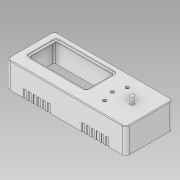
# Autodesk Inventor part: TAPA SUPEIOR
Saved by Autodesk Inventor 2019 (Build 230136000, 136)
## iProperties
Created: 2019-07-31
Part Number: TAPA SUPEIOR
Material: Plástico ABS
Document SubType Name: Modeling
Designer: Luis Pujol
Density: 1.06 g/cm^3
Appearance: Suave - Blanco
Author: Luis Pujol
Autodesk Inventor part; units mm, degrees
ref_plane "YZ Plane" through (0, 0, 0) normal (1, 0, 0) x (0, 1, 0)
ref_plane "XZ Plane" through (0, 0, 0) normal (0, 1, 0) x (-1, 0, 0)
ref_plane "XY Plane" through (0, 0, 0) normal (0, 0, 1) x (1, 0, 0)
sketch "Boceto1" plane through (0, 0, 0) normal (0, 1, 0) x (-1, 0, 0)
  line L0 (87.5, 35) -> (-87.5, 35)
  line L1 (-87.5, 35) -> (-87.5, -35)
  line L2 (-87.5, -35) -> (87.5, -35)
  line L3 (87.5, -35) -> (87.5, 35)
  line L4 (87.5, 35) -> (-87.5, -35) construction
  line L5 (-87.5, 35) -> (87.5, -35) construction
  point P0 (0, 0)
  dimension "d0" = 175
  dimension "d1" = 70
  constraints: 12 end point, 2 midpoint, 2 parallel, 1 horizontal, 1 perpendicular
  measures "d0" distance of L2.end L1.end
  measures "d1" distance of L1.end L0.end
extrude "Extrusión1" add sketch "Boceto1" along normal blind 2.8
fillet "Empalme1" radius 5 4 edges at (87.5, 1.4, 35) (87.5, 1.4, -35) (-87.5, 1.4, 35) (-87.5, 1.4, -35)
sketch "Boceto2" plane through (0, 0, 0) normal (0, -1, 0) x (1, 0, 0)
  arc A0 (-87.5, -30) -> (-82.5, -35) centre (-82.5, -30) ccw projected
  line L0 (82.5, -35) -> (-82.5, -35) projected
  arc A1 (82.5, -35) -> (87.5, -30) centre (82.5, -30) ccw projected
  line L1 (87.5, 30) -> (87.5, -30) projected
  arc A2 (87.5, 30) -> (82.5, 35) centre (82.5, 30) ccw projected
  line L2 (-82.5, 35) -> (82.5, 35) projected
  arc A3 (-82.5, 35) -> (-87.5, 30) centre (-82.5, 30) ccw projected
  line L3 (-87.5, -30) -> (-87.5, 30) projected
  arc A4 (84.7, 30) -> (82.5, 32.2) centre (82.5, 30) ccw
  line L4 (84.7, 30) -> (84.7, -30)
  arc A5 (82.5, -32.2) -> (84.7, -30) centre (82.5, -30) ccw
  line L5 (82.5, -32.2) -> (-82.5, -32.2)
  arc A6 (-84.7, -30) -> (-82.5, -32.2) centre (-82.5, -30) ccw
  line L6 (-84.7, -30) -> (-84.7, 30)
  arc A7 (-82.5, 32.2) -> (-84.7, 30) centre (-82.5, 30) ccw
  line L7 (-82.5, 32.2) -> (82.5, 32.2)
  point P0 (0, 0)
  dimension "d5" = 2.8
  constraints: 8 end point, 8 point on circle, 4 centre point, 7 other
  measures "d5" distance between parallel lines of L2 L7
extrude "Extrusión2" add sketch "Boceto2" along normal blind 35
sketch "Boceto8" plane through (0, 0, 0) normal (0, -1, 0) x (1, 0, 0)
  circle A0 centre (24.3039, 17.2337) radius 2.5
  point P0 (0, 0)
  dimension "d40" = 5
  constraints: 1 centre point
  measures "d40" diameter of A0
extrude "Extrusión8" add sketch "Boceto8" along normal blind 3.3
fillet "Empalme3" radius 0.5 2 edges at (21.8039, 0, 17.2337) (21.8039, -3.3, 17.2337)
sketch "Boceto11" plane through (24.3039, -3.3, 17.2337) normal (0, -1, 0) x (1, 0, 0)
  circle A0 centre (0, 0) radius 2 projected
  point P0 (-24.3039, -17.2337)
hole "Agujero2" at (24.3039, -3.3, 17.2337) direction (0, 1, 0) diameter 1.8 depth 5 tip angle 118 countersink diameter 2.5 countersink angle 90
fillet "Empalme4" radius 1 8 edges at (-86.0355, 2.8, 33.5355) (0, 2.8, 35) (86.0355, 2.8, 33.5355) (87.5, 2.8, 0) (86.0355, 2.8, -33.5355) (0, 2.8, -35) (-86.0355, 2.8, -33.5355) (-87.5, 2.8, 0)
sketch "Boceto14" plane through (0, 2.8, 0) normal (0, 1, 0) x (1, 0, 0)
  line L0 (-77.5, -18) -> (12.5, -18)
  line L1 (12.5, -18) -> (12.5, 28)
  line L2 (12.5, 28) -> (-77.5, 28)
  line L3 (-77.5, 28) -> (-77.5, -18)
  line L4 (-77.5, -18) -> (12.5, 28) construction
  line L5 (12.5, -18) -> (-77.5, 28) construction
  line L6 (-87.5, 30) -> (-87.5, -30) projected
  line L7 (82.5, -34) -> (-82.5, -34) projected
  point P0 (0, 0)
  point P1 (-32.5, 5)
  dimension "d69" = 90
  dimension "d70" = 46
  dimension "d71" = 55
  dimension "d72" = 16
  constraints: 12 end point, 2 midpoint, 2 parallel, 1 horizontal, 1 perpendicular
  measures "d69" distance of L2.end L1.end
  measures "d70" distance of L1.end L0.end
  measures "d71" distance from line of L6 point (-32.5, 5)
  measures "d72" distance between parallel lines of L7 L0
extrude "Extrusión10" cut sketch "Boceto14" against normal blind 1.5
fillet "Empalme6" radius 5 4 edges at (-77.5, 2.05, -28) (12.5, 2.05, -28) (12.5, 2.05, 18) (-77.5, 2.05, 18)
sketch "Boceto15" plane through (0, 1.3, 0) normal (0, 1, 0) x (1, 0, 0)
  line L0 (12.5, 23) -> (12.5, -13) projected
  arc A0 (7.5, -18) -> (12.5, -13) centre (7.5, -13) ccw projected
  line L1 (7.5, -18) -> (-72.5, -18) projected
  arc A1 (-77.5, -13) -> (-72.5, -18) centre (-72.5, -13) ccw projected
  line L2 (-77.5, -13) -> (-77.5, 23) projected
  arc A2 (-72.5, 28) -> (-77.5, 23) centre (-72.5, 23) ccw projected
  line L3 (-72.5, 28) -> (7.5, 28) projected
  arc A3 (12.5, 23) -> (7.5, 28) centre (7.5, 23) ccw projected
  arc A4 (-86.5, -30) -> (-82.5, -34) centre (-82.5, -30) ccw projected
  line L4 (82.5, -34) -> (-82.5, -34) projected
  arc A5 (82.5, -34) -> (86.5, -30) centre (82.5, -30) ccw projected
  line L5 (86.5, 30) -> (86.5, -30) projected
  arc A6 (86.5, 30) -> (82.5, 34) centre (82.5, 30) ccw projected
  line L6 (-82.5, 34) -> (82.5, 34) projected
  arc A7 (-82.5, 34) -> (-86.5, 30) centre (-82.5, 30) ccw projected
  line L7 (-86.5, -30) -> (-86.5, 30) projected
  line L8 (7.5, 25.2) -> (-72.5, 25.2)
  arc A8 (-72.5, 25.2) -> (-74.7, 23) centre (-72.5, 23) ccw
  line L9 (-74.7, 23) -> (-74.7, -13)
  arc A9 (-74.7, -13) -> (-72.5, -15.2) centre (-72.5, -13) ccw
  line L10 (-72.5, -15.2) -> (7.5, -15.2)
  arc A10 (7.5, -15.2) -> (9.7, -13) centre (7.5, -13) ccw
  line L11 (9.7, -13) -> (9.7, 23)
  arc A11 (9.7, 23) -> (7.5, 25.2) centre (7.5, 23) ccw
  point P0 (0, 0)
  dimension "d76" = 2.8
  constraints: 8 end point, 8 point on circle, 4 centre point, 7 other
  measures "d76" distance between parallel lines of L3 L8
extrude "Extrusión11" cut sketch "Boceto15" against normal blind 1.5 contours A11 L11 A10 L10 A9 L9 A8 L8
sketch "Boceto16" plane through (-82.5, -35, 35) normal (0, 0, 1) x (1, 0, 0)
  line L0 (0, 36.8) -> (165, 36.8) projected
  line L1 (0, 36.8) -> (0, 0) projected
  line L2 (165, 0) -> (0, 0) projected
  line L3 (165, 36.8) -> (165, 0) projected
  line L4 (55, 0) -> (59.2857, 0)
  line L5 (59.2857, 0) -> (59.2857, 12)
  line L6 (59.2857, 12) -> (55, 12)
  line L7 (55, 12) -> (55, 0)
  line L8 (55, 0) -> (59.2857, 12) construction
  line L9 (59.2857, 0) -> (55, 12) construction
  point P0 (82.5, 35)
  point P1 (57.1429, 6)
  point P2 (57.1429, 0)
  constraints: 12 end point, 3 midpoint, 2 parallel, 1 horizontal, 1 horizontal alignment, 1 perpendicular
extrude "Extrusión12" cut sketch "Boceto16" against normal blind 1 contours L7 L6 L5 L2
sketch "Boceto17" plane through (-82.5, 1.8, 35) normal (0, 0, 1) x (1, 0, 0)
  line L0 (55, -36.8) -> (55, -24.8) projected
  line L1 (55, -24.8) -> (59.2857, -24.8) projected
  line L2 (59.2857, -24.8) -> (59.2857, -36.8) projected
  line L3 (165, -36.8) -> (59.2857, -36.8) projected
  line L4 (165, 0) -> (165, -36.8) projected
  line L5 (0, 0) -> (165, 0) projected
  line L6 (0, 0) -> (0, -36.8) projected
  line L7 (55, -36.8) -> (0, -36.8) projected
  line L8 (105.732, -36.8) -> (110, -36.8)
  line L9 (110, -36.8) -> (110, -24.8)
  line L10 (110, -24.8) -> (105.732, -24.8)
  line L11 (105.732, -24.8) -> (105.732, -36.8)
  line L12 (105.732, -36.8) -> (110, -24.8) construction
  line L13 (110, -36.8) -> (105.732, -24.8) construction
  point P0 (82.5, -1.8)
  point P1 (107.866, -30.8)
  dimension "d83" = 4.268
  constraints: 12 end point, 2 midpoint, 2 parallel, 1 horizontal, 1 perpendicular
  measures "d83" distance of L9.end L10.end
extrude "Extrusión13" cut sketch "Boceto17" against normal blind 1 contours L11 L10 L9 L3
pattern_linear "Patrón rectangular1" count 6 spacing 7 along (-1, 0, 0) of "Extrusión12"
pattern_linear "Patrón rectangular2" count 6 spacing 7 along (1, 0, 0) of "Extrusión13"
mirror "Simetría1" about plane through (0, 0, 0) normal (0, 0, 1) of "Extrusión12", "Patrón rectangular1", "Extrusión13", "Patrón rectangular2"
sketch "Boceto18" plane through (0, 2.8, 0) normal (0, 1, 0) x (1, 0, 0)
  circle A0 centre (62, 0) radius 3
  circle A1 centre (62, 0) radius 29 construction
  circle A2 centre (33, 0) radius 2.5
  circle A3 centre (38.2446, 16.6337) radius 2.5
  circle A4 centre (38.2446, -16.6337) radius 2.5
  point P0 (0, 0)
  dimension "d92" = 6
  dimension "d95" = 35
  dimension "d97" = 5
  dimension "d98" = 5
  dimension "d99" = 5
  constraints: 5 centre point, 4 coincident, 2 point on circle, 2 other
  measures "d92" diameter of A0
  measures "d97" diameter of A2
  measures "d98" diameter of A3
  measures "d99" diameter of A4
extrude "Extrusión14" cut sketch "Boceto18" against normal blind 5
sketch "Boceto19" plane through (0, 2.8, 0) normal (0, 1, 0) x (1, 0, 0)
  circle A0 centre (38.2446, -16.6337) radius 2.5 projected
  circle A1 centre (33, 0) radius 2.5 projected
  circle A2 centre (38.2446, 16.6337) radius 2.5 projected
  circle A3 centre (62, 0) radius 3 projected
  line L0 (12.5, 23) -> (12.5, -13) projected
  arc A4 (7.5, -18) -> (12.5, -13) centre (7.5, -13) ccw projected
  line L1 (7.5, -18) -> (-72.5, -18) projected
  arc A5 (-77.5, -13) -> (-72.5, -18) centre (-72.5, -13) ccw projected
  line L2 (-77.5, -13) -> (-77.5, 23) projected
  arc A6 (-72.5, 28) -> (-77.5, 23) centre (-72.5, 23) ccw projected
  line L3 (-72.5, 28) -> (7.5, 28) projected
  arc A7 (12.5, 23) -> (7.5, 28) centre (7.5, 23) ccw projected
  arc A8 (-86.5, -30) -> (-82.5, -34) centre (-82.5, -30) ccw projected
  line L4 (82.5, -34) -> (-82.5, -34) projected
  arc A9 (82.5, -34) -> (86.5, -30) centre (82.5, -30) ccw projected
  line L5 (86.5, 30) -> (86.5, -30) projected
  arc A10 (86.5, 30) -> (82.5, 34) centre (82.5, 30) ccw projected
  line L6 (-82.5, 34) -> (82.5, 34) projected
  arc A11 (-82.5, 34) -> (-86.5, 30) centre (-82.5, 30) ccw projected
  line L7 (-86.5, -30) -> (-86.5, 30) projected
  circle A12 centre (62, 0) radius 3 projected
  circle A13 centre (62, 0) radius 3
  point P0 (0, 0)
  constraints: 1 centre point, 1 coincident
extrude "Extrusión15" add sketch "Boceto19" along normal blind 10 contours A3
